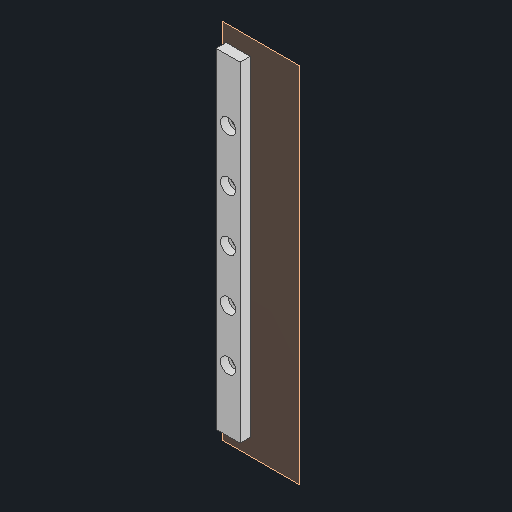
# Autodesk Inventor part: pci_slot_adapter_02
Saved by Autodesk Inventor 2022 (Build 260153000, 153)
## iProperties
Created: 2025-02-02
Part Number: pci_slot_adapter_02
Material: 一般
Document SubType Name: Modeling
Designer: nyxeon
Density: 1 g/cm^3
Appearance: 既定
Author: nyxeon
Autodesk Inventor part; units mm, degrees
ref_plane "YZ Plane" through (0, 0, 0) normal (1, 0, 0) x (0, 1, 0)
ref_plane "XZ Plane" through (0, 0, 0) normal (0, 1, 0) x (-1, 0, 0)
ref_plane "XY Plane" through (0, 0, 0) normal (0, 0, 1) x (1, 0, 0)
ref_plane "作業平面1" through (0, 0, 0) normal (0, 0, 1) x (1, 0, 0)
sketch "スケッチ1" plane through (0, 0, 0) normal (0, 0, 1) x (1, 0, 0)
  circle A0 centre (-2.4335, -0.0165) radius 2.25 construction
  circle A1 centre (-2.4335, 20.4165) radius 2.25 construction
  circle A2 centre (-2.4335, -20.4495) radius 2.25 construction
  circle A3 centre (-2.4335, 40.8495) radius 2.25 construction
  circle A4 centre (-2.4335, -40.8824) radius 2.25 construction
  arc A5 (7.0535, -60.5275) -> (7.932, -61.0497) centre (7.932, -60.0497) ccw construction
  arc A6 (7.0535, -60.5275) -> (6.8807, -60.2968) centre (6.175, -61.0052) ccw construction
  line L0 (6.8807, -60.2968) -> (2.9106, -56.342) construction
  arc A7 (2.9106, -56.342) -> (2.8353, -56.3081) centre (2.8355, -56.4081) ccw construction
  line L1 (2.8353, -56.3081) -> (-2.8421, -56.3081) construction
  arc A8 (-4.2232, -54.98) -> (-2.8421, -56.3081) centre (-2.825, -54.9082) ccw construction
  line L2 (-4.2232, -54.98) -> (-4.2232, -46.9628) construction
  arc A9 (-2.825, -45.4911) -> (-4.2232, -46.9628) centre (-2.825, -46.8911) ccw construction
  line L3 (-2.825, -45.4911) -> (2.8507, -45.4911) construction
  arc A10 (2.8507, -45.4911) -> (2.9214, -45.4618) centre (2.8507, -45.3911) ccw construction
  line L4 (2.9214, -45.4618) -> (6.8821, -41.5011) construction
  arc A11 (6.8821, -41.5011) -> (7.175, -40.794) centre (6.175, -40.794) ccw construction
  line L5 (7.175, -40.794) -> (7.175, -40.7051) construction
  arc A12 (7.175, -40.7051) -> (6.8821, -39.998) centre (6.175, -40.7051) ccw construction
  line L6 (6.8821, -39.998) -> (2.9214, -36.0374) construction
  arc A13 (2.9214, -36.0374) -> (2.8507, -36.0081) centre (2.8507, -36.1081) ccw construction
  line L7 (2.8507, -36.0081) -> (-2.825, -36.0081) construction
  arc A14 (-4.225, -34.6081) -> (-2.825, -36.0081) centre (-2.825, -34.6081) ccw construction
  line L8 (-4.225, -34.6081) -> (-4.225, -26.4581) construction
  arc A15 (-2.825, -25.0581) -> (-4.225, -26.4581) centre (-2.825, -26.4581) ccw construction
  line L9 (-2.825, -25.0581) -> (2.8507, -25.0581) construction
  arc A16 (2.8507, -25.0581) -> (2.9214, -25.0288) centre (2.8507, -24.9581) ccw construction
  line L10 (2.9214, -25.0288) -> (6.8821, -21.0681) construction
  arc A17 (6.8821, -21.0681) -> (7.175, -20.361) centre (6.175, -20.361) ccw construction
  line L11 (7.175, -20.361) -> (7.175, -20.2722) construction
  arc A18 (7.175, -20.2722) -> (6.8807, -19.5637) centre (6.175, -20.2722) ccw construction
  line L12 (6.8807, -19.5637) -> (2.9106, -15.609) construction
  arc A19 (2.9106, -15.609) -> (2.8353, -15.575) centre (2.8355, -15.675) ccw construction
  line L13 (2.8353, -15.575) -> (-2.8421, -15.575) construction
  arc A20 (-4.2232, -14.2469) -> (-2.8421, -15.575) centre (-2.825, -14.1751) ccw construction
  line L14 (-4.2232, -14.2469) -> (-4.2232, -6.2297) construction
  arc A21 (-2.825, -4.758) -> (-4.2232, -6.2297) centre (-2.825, -6.158) ccw construction
  line L15 (-2.825, -4.758) -> (2.8507, -4.758) construction
  arc A22 (2.8507, -4.758) -> (2.9214, -4.7287) centre (2.8507, -4.658) ccw construction
  line L16 (2.9214, -4.7287) -> (6.8821, -0.768) construction
  arc A23 (6.8821, -0.768) -> (7.175, -0.0609) centre (6.175, -0.0609) ccw construction
  line L17 (7.175, -0.0609) -> (7.175, 0.0279) construction
  arc A24 (7.175, 0.0279) -> (6.8821, 0.7351) centre (6.175, 0.0279) ccw construction
  line L18 (6.8821, 0.7351) -> (2.9214, 4.6957) construction
  arc A25 (2.9214, 4.6957) -> (2.8507, 4.725) centre (2.8507, 4.625) ccw construction
  line L19 (2.8507, 4.725) -> (-2.825, 4.725) construction
  arc A26 (-4.225, 6.125) -> (-2.825, 4.725) centre (-2.825, 6.125) ccw construction
  line L20 (-4.225, 6.125) -> (-4.225, 14.275) construction
  arc A27 (-2.825, 15.675) -> (-4.225, 14.275) centre (-2.825, 14.275) ccw construction
  line L21 (-2.825, 15.675) -> (2.8507, 15.675) construction
  arc A28 (2.8507, 15.675) -> (2.9214, 15.7043) centre (2.8507, 15.775) ccw construction
  line L22 (2.9214, 15.7043) -> (6.8821, 19.6649) construction
  arc A29 (6.8821, 19.6649) -> (7.175, 20.3721) centre (6.175, 20.3721) ccw construction
  line L23 (7.175, 20.3721) -> (7.175, 20.4609) construction
  arc A30 (7.175, 20.4609) -> (6.8821, 21.168) centre (6.175, 20.4609) ccw construction
  line L24 (6.8821, 21.168) -> (2.9214, 25.1287) construction
  arc A31 (2.9214, 25.1287) -> (2.8507, 25.158) centre (2.8507, 25.058) ccw construction
  line L25 (2.8507, 25.158) -> (-2.825, 25.158) construction
  arc A32 (-4.2232, 26.6297) -> (-2.825, 25.158) centre (-2.825, 26.558) ccw construction
  line L26 (-4.2232, 26.6297) -> (-4.2232, 34.6469) construction
  arc A33 (-2.8421, 35.975) -> (-4.2232, 34.6469) centre (-2.825, 34.5751) ccw construction
  line L27 (-2.8421, 35.975) -> (2.8353, 35.975) construction
  arc A34 (2.8353, 35.975) -> (2.9106, 36.009) centre (2.8355, 36.075) ccw construction
  line L28 (2.9106, 36.009) -> (6.8807, 39.9637) construction
  arc A35 (6.8807, 39.9637) -> (7.175, 40.6722) centre (6.175, 40.6722) ccw construction
  line L29 (7.175, 40.6722) -> (7.175, 40.761) construction
  arc A36 (7.175, 40.761) -> (6.8821, 41.4681) centre (6.175, 40.761) ccw construction
  line L30 (6.8821, 41.4681) -> (2.9214, 45.4288) construction
  arc A37 (2.9214, 45.4288) -> (2.8507, 45.4581) centre (2.8507, 45.3581) ccw construction
  line L31 (2.8507, 45.4581) -> (-2.825, 45.4581) construction
  arc A38 (-4.225, 46.8581) -> (-2.825, 45.4581) centre (-2.825, 46.8581) ccw construction
  line L32 (-4.225, 46.8581) -> (-4.225, 55.0081) construction
  arc A39 (-2.825, 56.4081) -> (-4.225, 55.0081) centre (-2.825, 55.0081) ccw construction
  line L33 (-2.825, 56.4081) -> (2.8507, 56.4081) construction
  arc A40 (2.8507, 56.4081) -> (2.9214, 56.4374) centre (2.8507, 56.5081) ccw construction
  line L34 (2.9214, 56.4374) -> (6.8821, 60.398) construction
  arc A41 (6.8821, 60.398) -> (7.0535, 60.6274) centre (6.175, 61.1051) ccw construction
  arc A42 (7.932, 61.1496) -> (7.0535, 60.6274) centre (7.932, 60.1496) ccw construction
  line L35 (7.932, 61.1496) -> (20.325, 61.1496) construction
  line L36 (20.325, 61.1496) -> (20.325, 65) construction
  line L37 (20.325, 65) -> (-7.175, 65) construction
  line L38 (-7.175, 65) -> (-7.175, -65) construction
  line L39 (-7.175, -65) -> (20.325, -65) construction
  line L40 (20.325, -65) -> (20.325, -61.0497) construction
  line L41 (20.325, -61.0497) -> (7.932, -61.0497) construction
  circle A43 centre (-2.4335, 40.8495) radius 1.65
  circle A44 centre (-2.4335, 20.4165) radius 1.65
  circle A45 centre (-2.4335, -0.0165) radius 1.65
  circle A46 centre (-2.4335, -20.4495) radius 1.65
  circle A47 centre (-2.4335, -40.8824) radius 1.65
  line L42 (-7.175, 65) -> (2.308, 65)
  line L43 (2.308, 65) -> (2.308, -65)
  line L44 (2.308, -65) -> (-7.175, -65)
  line L45 (-7.175, -65) -> (-7.175, 65)
  point P0 (0, 0)
  dimension "d0" = 3.3
  dimension "d1" = 4.7415
  dimension "d2" = 4.7415
  constraints: 8 end point, 5 centre point, 5 coincident, 4 equal radius, 2 parallel, 1 horizontal, 1 perpendicular, 1 point on line
  measures "d0" diameter of A43
  measures "d1" distance from line of L38 A3.centre
  measures "d2" distance from line of A3.centre L43
extrude "押し出し1" add sketch "スケッチ1" along normal blind 4
sketch "スケッチ2" plane through (0, 0, 4) normal (0, 0, 1) x (1, 0, 0)
  circle A0 centre (-2.4335, 40.8495) radius 1.65 construction
  circle A1 centre (-2.4335, 20.4165) radius 1.65 construction
  circle A2 centre (-2.4335, -0.0165) radius 1.65 construction
  circle A3 centre (-2.4335, -20.4495) radius 1.65 construction
  circle A4 centre (-2.4335, -40.8824) radius 1.65 construction
  circle A5 centre (-2.4335, 40.8495) radius 1.65 projected
  circle A6 centre (-2.4335, 40.8495) radius 3
  circle A7 centre (-2.4335, 20.4165) radius 3
  circle A8 centre (-2.4335, -0.0165) radius 3
  circle A9 centre (-2.4335, -20.4495) radius 1.65 projected
  circle A10 centre (-2.4335, -20.4495) radius 3
  circle A11 centre (-2.4335, -40.8824) radius 3
  point P0 (0, 0)
  dimension "d5" = 6
  constraints: 5 centre point, 5 coincident, 4 equal radius
  measures "d5" diameter of A6
extrude "押し出し2" cut sketch "スケッチ2" against normal blind 3
equation "\"d2\" = d1"
